Autodesk Fusion 360 part; units mm, degrees
(part 5 of 12)
  line L806 (6.8281, 44.0008) -> (6.6464, 43.7508)
  line L807 (6.8281, 44.3098) -> (6.8281, 44.0008)
  line L808 (6.3475, 43.6553) -> (6.0536, 43.7508)
  line L809 (6.3526, 44.6553) -> (6.6464, 44.5598)
  line L810 (6.3475, 44.6553) -> (6.3526, 44.6553)
  line L811 (6.0536, 44.5598) -> (6.3475, 44.6553)
  line L812 (6.0536, 43.7508) -> (5.8719, 44.0008)
  line L813 (5.8719, 44.3098) -> (6.0536, 44.5598)
  line L814 (6.3475, 41.1153) -> (6.0536, 41.2108)
  line L815 (6.0536, 41.2108) -> (5.8719, 41.4608)
  line L816 (5.8719, 41.4608) -> (5.8719, 41.7698)
  line L817 (5.8719, 41.7698) -> (6.0536, 42.0198)
  line L818 (6.0536, 42.0198) -> (6.3475, 42.1153)
  line L819 (6.3475, 42.1153) -> (6.3526, 42.1153)
  line L820 (6.3526, 42.1153) -> (6.6464, 42.0198)
  line L821 (6.6464, 42.0198) -> (6.8281, 41.7698)
  line L822 (6.8281, 41.7698) -> (6.8281, 41.4608)
  line L823 (6.8281, 41.4608) -> (6.6464, 41.2108)
  line L824 (6.6464, 41.2108) -> (6.3526, 41.1153)
  line L825 (6.3526, 41.1153) -> (6.3475, 41.1153)
  line L826 (5.8719, 39.2298) -> (6.0536, 39.4798)
  line L827 (5.8719, 38.9208) -> (5.8719, 39.2298)
  line L828 (6.3475, 38.5753) -> (6.0536, 38.6708)
  line L829 (6.0536, 39.4798) -> (6.3475, 39.5753)
  line L830 (6.3475, 39.5753) -> (6.3526, 39.5753)
  line L831 (6.3526, 39.5753) -> (6.6464, 39.4798)
  line L832 (6.6464, 39.4798) -> (6.8281, 39.2298)
  line L833 (6.8281, 39.2298) -> (6.8281, 38.9208)
  line L834 (6.8281, 38.9208) -> (6.6464, 38.6708)
  line L835 (6.6464, 38.6708) -> (6.3526, 38.5753)
  line L836 (6.3526, 38.5753) -> (6.3475, 38.5753)
  line L837 (6.0536, 38.6708) -> (5.8719, 38.9208)
  line L838 (23.8336, 39.4798) -> (24.1275, 39.5753)
  line L839 (24.1326, 39.5753) -> (24.4265, 39.4798)
  line L840 (23.8336, 38.6708) -> (23.652, 38.9208)
  line L841 (24.1275, 38.5753) -> (23.8336, 38.6708)
  line L842 (24.4265, 39.4798) -> (24.6081, 39.2298)
  line L843 (24.6081, 39.2298) -> (24.6081, 38.9208)
  line L844 (24.6081, 38.9208) -> (24.4265, 38.6708)
  line L845 (24.4265, 38.6708) -> (24.1326, 38.5753)
  line L846 (24.1326, 38.5753) -> (24.1275, 38.5753)
  line L847 (23.652, 39.2298) -> (23.8336, 39.4798)
  line L848 (24.1275, 39.5753) -> (24.1326, 39.5753)
  line L849 (23.652, 38.9208) -> (23.652, 39.2298)
  line L850 (24.1275, 41.1153) -> (23.8336, 41.2108)
  line L851 (23.8336, 41.2108) -> (23.652, 41.4608)
  line L852 (23.652, 41.4608) -> (23.652, 41.7698)
  line L853 (23.652, 41.7698) -> (23.8336, 42.0198)
  line L854 (23.8336, 42.0198) -> (24.1275, 42.1153)
  line L855 (24.1275, 42.1153) -> (24.1326, 42.1153)
  line L856 (24.1326, 42.1153) -> (24.4265, 42.0198)
  line L857 (24.4265, 42.0198) -> (24.6081, 41.7698)
  line L858 (24.6081, 41.7698) -> (24.6081, 41.4608)
  line L859 (24.6081, 41.4608) -> (24.4265, 41.2108)
  line L860 (24.4265, 41.2108) -> (24.1326, 41.1153)
  line L861 (24.1326, 41.1153) -> (24.1275, 41.1153)
  line L862 (23.652, 43.9292) -> (23.652, 44.2382)
  line L863 (23.652, 44.2382) -> (23.8336, 44.4882)
  line L864 (23.8336, 44.4882) -> (24.1275, 44.5837)
  line L865 (24.1275, 44.5837) -> (24.1326, 44.5837)
  line L866 (24.1326, 44.5837) -> (24.4265, 44.4882)
  line L867 (23.8336, 43.6792) -> (23.652, 43.9292)
  line L868 (24.1275, 43.5837) -> (23.8336, 43.6792)
  line L869 (24.4265, 44.4882) -> (24.6081, 44.2382)
  line L870 (24.6081, 44.2382) -> (24.6081, 43.9292)
  line L871 (24.6081, 43.9292) -> (24.4265, 43.6792)
  line L872 (24.4265, 43.6792) -> (24.1326, 43.5837)
  line L873 (24.1326, 43.5837) -> (24.1275, 43.5837)
  line L874 (24.1275, 46.1953) -> (23.8336, 46.2908)
  line L875 (24.1326, 46.1953) -> (24.1275, 46.1953)
  line L876 (24.4265, 46.2908) -> (24.1326, 46.1953)
  line L877 (24.6081, 46.5408) -> (24.4265, 46.2908)
  line L878 (24.6081, 46.8498) -> (24.6081, 46.5408)
  line L879 (24.4265, 47.0998) -> (24.6081, 46.8498)
  line L880 (24.1326, 47.1953) -> (24.4265, 47.0998)
  line L881 (24.1275, 47.1953) -> (24.1326, 47.1953)
  line L882 (23.8336, 47.0998) -> (24.1275, 47.1953)
  line L883 (23.652, 46.8498) -> (23.8336, 47.0998)
  line L884 (23.652, 46.5408) -> (23.652, 46.8498)
  line L885 (23.8336, 46.2908) -> (23.652, 46.5408)
  line L886 (24.1326, 48.7353) -> (24.1275, 48.7353)
  line L887 (24.1275, 48.7353) -> (23.8336, 48.8308)
  line L888 (23.8336, 48.8308) -> (23.652, 49.0808)
  line L889 (23.652, 49.0808) -> (23.652, 49.3898)
  line L890 (23.652, 49.3898) -> (23.8336, 49.6398)
  line L891 (23.8336, 49.6398) -> (24.1275, 49.7353)
  line L892 (24.1275, 49.7353) -> (24.1326, 49.7353)
  line L893 (24.4265, 49.6398) -> (24.6081, 49.3898)
  line L894 (24.6081, 49.3898) -> (24.6081, 49.0808)
  line L895 (24.6081, 49.0808) -> (24.4265, 48.8308)
  line L896 (24.4265, 48.8308) -> (24.1326, 48.7353)
  line L897 (24.1326, 49.7353) -> (24.4265, 49.6398)
  line L898 (24.1326, 52.2753) -> (24.4265, 52.1798)
  line L899 (24.1275, 51.2753) -> (23.8336, 51.3708)
  line L900 (23.8336, 51.3708) -> (23.652, 51.6208)
  line L901 (23.652, 51.6208) -> (23.652, 51.9298)
  line L902 (23.652, 51.9298) -> (23.8336, 52.1798)
  line L903 (23.8336, 52.1798) -> (24.1275, 52.2753)
  line L904 (24.1275, 52.2753) -> (24.1326, 52.2753)
  line L905 (24.1326, 51.2753) -> (24.1275, 51.2753)
  line L906 (24.4265, 51.3708) -> (24.1326, 51.2753)
  line L907 (24.6081, 51.6208) -> (24.4265, 51.3708)
  line L908 (24.6081, 51.9298) -> (24.6081, 51.6208)
  line L909 (24.4265, 52.1798) -> (24.6081, 51.9298)
  line L910 (24.1326, 53.8153) -> (24.1275, 53.8153)
  line L911 (24.4265, 53.9108) -> (24.1326, 53.8153)
  line L912 (24.6081, 54.1608) -> (24.4265, 53.9108)
  line L913 (24.6081, 54.4698) -> (24.6081, 54.1608)
  line L914 (24.4265, 54.7198) -> (24.6081, 54.4698)
  line L915 (23.652, 54.4698) -> (23.8336, 54.7198)
  line L916 (23.652, 54.1608) -> (23.652, 54.4698)
  line L917 (23.8336, 53.9108) -> (23.652, 54.1608)
  line L918 (24.1275, 53.8153) -> (23.8336, 53.9108)
  line L919 (24.1326, 54.8153) -> (24.4265, 54.7198)
  line L920 (23.8336, 54.7198) -> (24.1275, 54.8153)
  line L921 (24.1275, 54.8153) -> (24.1326, 54.8153)
  line L922 (24.1275, 57.3553) -> (24.1326, 57.3553)
  line L923 (24.1326, 57.3553) -> (24.4265, 57.2598)
  line L924 (23.8336, 57.2598) -> (24.1275, 57.3553)
  line L925 (24.1275, 56.3553) -> (23.8336, 56.4508)
  line L926 (23.8336, 56.4508) -> (23.652, 56.7008)
  line L927 (23.652, 56.7008) -> (23.652, 57.0098)
  line L928 (23.652, 57.0098) -> (23.8336, 57.2598)
  line L929 (24.4265, 57.2598) -> (24.6081, 57.0098)
  line L930 (24.6081, 57.0098) -> (24.6081, 56.7008)
  line L931 (24.6081, 56.7008) -> (24.4265, 56.4508)
  line L932 (24.4265, 56.4508) -> (24.1326, 56.3553)
  line L933 (24.1326, 56.3553) -> (24.1275, 56.3553)
  line L934 (24.1326, 59.8953) -> (24.4265, 59.7998)
  line L935 (23.8336, 58.9908) -> (23.652, 59.2408)
  line L936 (23.652, 59.2408) -> (23.652, 59.5498)
  line L937 (23.652, 59.5498) -> (23.8336, 59.7998)
  line L938 (23.8336, 59.7998) -> (24.1275, 59.8953)
  line L939 (24.1275, 59.8953) -> (24.1326, 59.8953)
  line L940 (24.1275, 58.8953) -> (23.8336, 58.9908)
  line L941 (24.4265, 59.7998) -> (24.6081, 59.5498)
  line L942 (24.6081, 59.5498) -> (24.6081, 59.2408)
  line L943 (24.6081, 59.2408) -> (24.4265, 58.9908)
  line L944 (24.4265, 58.9908) -> (24.1326, 58.8953)
  line L945 (24.1326, 58.8953) -> (24.1275, 58.8953)
  line L946 (24.1275, 61.4353) -> (23.8336, 61.5308)
  line L947 (23.8336, 61.5308) -> (23.652, 61.7808)
  line L948 (23.652, 61.7808) -> (23.652, 62.0898)
  line L949 (23.652, 62.0898) -> (23.8336, 62.3398)
  line L950 (23.8336, 62.3398) -> (24.1275, 62.4353)
  line L951 (24.1275, 62.4353) -> (24.1326, 62.4353)
  line L952 (24.1326, 62.4353) -> (24.4265, 62.3398)
  line L953 (24.4265, 62.3398) -> (24.6081, 62.0898)
  line L954 (24.6081, 62.0898) -> (24.6081, 61.7808)
  line L955 (24.6081, 61.7808) -> (24.4265, 61.5308)
  line L956 (24.4265, 61.5308) -> (24.1326, 61.4353)
  line L957 (24.1326, 61.4353) -> (24.1275, 61.4353)
  line L958 (24.1326, 64.9753) -> (24.4265, 64.8798)
  line L959 (24.1326, 63.9753) -> (24.1275, 63.9753)
  line L960 (24.4265, 64.0708) -> (24.1326, 63.9753)
  line L961 (24.6081, 64.3208) -> (24.4265, 64.0708)
  line L962 (24.6081, 64.6298) -> (24.6081, 64.3208)
  line L963 (24.4265, 64.8798) -> (24.6081, 64.6298)
  line L964 (24.1275, 64.9753) -> (24.1326, 64.9753)
  line L965 (23.8336, 64.8798) -> (24.1275, 64.9753)
  line L966 (23.652, 64.6298) -> (23.8336, 64.8798)
  line L967 (23.652, 64.3208) -> (23.652, 64.6298)
  line L968 (23.8336, 64.0708) -> (23.652, 64.3208)
  line L969 (24.1275, 63.9753) -> (23.8336, 64.0708)
  line L970 (24.1275, 66.5153) -> (23.8336, 66.6108)
  line L971 (23.8336, 66.6108) -> (23.652, 66.8608)
  line L972 (23.652, 66.8608) -> (23.652, 67.1699)
  line L973 (23.652, 67.1699) -> (23.8336, 67.4199)
  line L974 (23.8336, 67.4199) -> (24.1275, 67.5153)
  line L975 (24.1275, 67.5153) -> (24.1326, 67.5153)
  line L976 (24.1326, 67.5153) -> (24.4265, 67.4199)
  line L977 (24.4265, 67.4199) -> (24.6081, 67.1699)
  line L978 (24.6081, 67.1699) -> (24.6081, 66.8608)
  line L979 (24.6081, 66.8608) -> (24.4265, 66.6108)
  line L980 (24.4265, 66.6108) -> (24.1326, 66.5153)
  line L981 (24.1326, 66.5153) -> (24.1275, 66.5153)
  line L982 (23.8336, 69.1508) -> (23.652, 69.4008)
  line L983 (23.652, 69.4008) -> (23.652, 69.7099)
  line L984 (23.652, 69.7099) -> (23.8336, 69.9599)
  line L985 (23.8336, 69.9599) -> (24.1275, 70.0553)
  line L986 (24.1275, 70.0553) -> (24.1326, 70.0553)
  line L987 (24.1326, 69.0553) -> (24.1275, 69.0553)
  line L988 (24.4265, 69.1508) -> (24.1326, 69.0553)
  line L989 (24.6081, 69.4008) -> (24.4265, 69.1508)
  line L990 (24.6081, 69.7099) -> (24.6081, 69.4008)
  line L991 (24.1275, 69.0553) -> (23.8336, 69.1508)
  line L992 (24.4265, 69.9599) -> (24.6081, 69.7099)
  line L993 (24.1326, 70.0553) -> (24.4265, 69.9599)
  line L994 (24.1326, 71.5954) -> (24.1275, 71.5954)
  line L995 (24.4265, 71.6908) -> (24.1326, 71.5954)
  line L996 (24.6081, 71.9408) -> (24.4265, 71.6908)
  line L997 (24.6081, 72.2499) -> (24.6081, 71.9408)
  line L998 (24.4265, 72.4999) -> (24.6081, 72.2499)
  line L999 (24.1326, 72.5954) -> (24.4265, 72.4999)
  line L1000 (24.1275, 72.5954) -> (24.1326, 72.5954)
  line L1001 (23.8336, 72.4999) -> (24.1275, 72.5954)
  line L1002 (23.652, 72.2499) -> (23.8336, 72.4999)
  line L1003 (23.652, 71.9408) -> (23.652, 72.2499)
  line L1004 (23.8336, 71.6908) -> (23.652, 71.9408)
  line L1005 (24.1275, 71.5954) -> (23.8336, 71.6908)
  line L1006 (24.6081, 74.7899) -> (24.6081, 74.4808)
  line L1007 (24.6081, 74.4808) -> (24.4265, 74.2308)
  line L1008 (24.4265, 75.0399) -> (24.6081, 74.7899)
  line L1009 (24.1275, 74.1354) -> (23.8336, 74.2308)
  line L1010 (23.8336, 74.2308) -> (23.652, 74.4808)
  line L1011 (23.652, 74.4808) -> (23.652, 74.7899)
  line L1012 (23.652, 74.7899) -> (23.8336, 75.0399)
  line L1013 (23.8336, 75.0399) -> (24.1275, 75.1354)
  line L1014 (24.1275, 75.1354) -> (24.1326, 75.1354)
  line L1015 (24.1326, 75.1354) -> (24.4265, 75.0399)
  line L1016 (24.4265, 74.2308) -> (24.1326, 74.1354)
  line L1017 (24.1326, 74.1354) -> (24.1275, 74.1354)
  line L1018 (24.1326, 76.6754) -> (24.1275, 76.6754)
  line L1019 (24.1275, 76.6754) -> (23.8336, 76.7709)
  line L1020 (23.8336, 76.7709) -> (23.652, 77.0209)
  line L1021 (23.652, 77.0209) -> (23.652, 77.3299)
  line L1022 (23.652, 77.3299) -> (23.8336, 77.5799)
  line L1023 (23.8336, 77.5799) -> (24.1275, 77.6754)
  line L1024 (24.1275, 77.6754) -> (24.1326, 77.6754)
  line L1025 (24.1326, 77.6754) -> (24.4265, 77.5799)
  line L1026 (24.4265, 77.5799) -> (24.6081, 77.3299)
  line L1027 (24.6081, 77.3299) -> (24.6081, 77.0209)
  line L1028 (24.6081, 77.0209) -> (24.4265, 76.7709)
  line L1029 (24.4265, 76.7709) -> (24.1326, 76.6754)
  line L1030 (24.1326, 79.2154) -> (24.1275, 79.2154)
  line L1031 (24.1275, 79.2154) -> (23.8336, 79.3109)
  line L1032 (23.8336, 79.3109) -> (23.652, 79.5609)
  line L1033 (23.652, 79.5609) -> (23.652, 79.8699)
  line L1034 (23.652, 79.8699) -> (23.8336, 80.1199)
  line L1035 (23.8336, 80.1199) -> (24.1275, 80.2154)
  line L1036 (24.1275, 80.2154) -> (24.1326, 80.2154)
  line L1037 (24.1326, 80.2154) -> (24.4265, 80.1199)
  line L1038 (24.4265, 80.1199) -> (24.6081, 79.8699)
  line L1039 (24.6081, 79.8699) -> (24.6081, 79.5609)
  line L1040 (24.6081, 79.5609) -> (24.4265, 79.3109)
  line L1041 (24.4265, 79.3109) -> (24.1326, 79.2154)
  line L1042 (23.652, 82.1009) -> (23.652, 82.4099)
  line L1043 (24.1275, 81.7554) -> (23.8336, 81.8509)
  line L1044 (23.652, 82.4099) -> (23.8336, 82.6599)
  line L1045 (23.8336, 81.8509) -> (23.652, 82.1009)
  line L1046 (23.8336, 82.6599) -> (24.1275, 82.7554)
  line L1047 (24.1275, 82.7554) -> (24.1326, 82.7554)
  line L1048 (24.1326, 82.7554) -> (24.4265, 82.6599)
  line L1049 (24.4265, 82.6599) -> (24.6081, 82.4099)
  line L1050 (24.6081, 82.4099) -> (24.6081, 82.1009)
  line L1051 (24.6081, 82.1009) -> (24.4265, 81.8509)
  line L1052 (24.4265, 81.8509) -> (24.1326, 81.7554)
  line L1053 (24.1326, 81.7554) -> (24.1275, 81.7554)
  line L1054 (24.1275, 84.2954) -> (23.8336, 84.3909)
  line L1055 (23.8336, 84.3909) -> (23.652, 84.6409)
  line L1056 (23.652, 84.6409) -> (23.652, 84.9499)
  line L1057 (23.652, 84.9499) -> (23.8336, 85.1999)
  line L1058 (23.8336, 85.1999) -> (24.1275, 85.2954)
  line L1059 (24.1275, 85.2954) -> (24.1326, 85.2954)
  line L1060 (24.1326, 85.2954) -> (24.4265, 85.1999)
  line L1061 (24.4265, 85.1999) -> (24.6081, 84.9499)
  line L1062 (24.6081, 84.9499) -> (24.6081, 84.6409)
  line L1063 (24.6081, 84.6409) -> (24.4265, 84.3909)
  line L1064 (24.4265, 84.3909) -> (24.1326, 84.2954)
  line L1065 (24.1326, 84.2954) -> (24.1275, 84.2954)
  line L1066 (24.1326, 87.8354) -> (24.4265, 87.7399)
  line L1067 (24.4265, 87.7399) -> (24.6081, 87.4899)
  line L1068 (24.1275, 86.8354) -> (23.8336, 86.9309)
  line L1069 (23.8336, 86.9309) -> (23.652, 87.1809)
  line L1070 (23.652, 87.1809) -> (23.652, 87.4899)
  line L1071 (23.652, 87.4899) -> (23.8336, 87.7399)
  line L1072 (23.8336, 87.7399) -> (24.1275, 87.8354)
  line L1073 (24.1275, 87.8354) -> (24.1326, 87.8354)
  line L1074 (24.6081, 87.1809) -> (24.4265, 86.9309)
  line L1075 (24.4265, 86.9309) -> (24.1326, 86.8354)
  line L1076 (24.1326, 86.8354) -> (24.1275, 86.8354)
  line L1077 (24.6081, 87.4899) -> (24.6081, 87.1809)
  line L1078 (11.4326, 38.5753) -> (11.4275, 38.5753)
  line L1079 (11.4275, 38.5753) -> (11.1336, 38.6708)
  line L1080 (11.1336, 38.6708) -> (10.952, 38.9208)
  line L1081 (10.952, 38.9208) -> (10.952, 39.2298)
  line L1082 (10.952, 39.2298) -> (11.1336, 39.4798)
  line L1083 (11.1336, 39.4798) -> (11.4275, 39.5753)
  line L1084 (11.4275, 39.5753) -> (11.4326, 39.5753)
  line L1085 (11.4326, 39.5753) -> (11.7265, 39.4798)
  line L1086 (11.7265, 39.4798) -> (11.9081, 39.2298)
  line L1087 (11.9081, 39.2298) -> (11.9081, 38.9208)
  line L1088 (11.9081, 38.9208) -> (11.7265, 38.6708)
  line L1089 (11.7265, 38.6708) -> (11.4326, 38.5753)
  line L1090 (14.2665, 39.4798) -> (14.4481, 39.2298)
  line L1091 (13.9726, 39.5753) -> (14.2665, 39.4798)
  line L1092 (13.9675, 39.5753) -> (13.9726, 39.5753)
  line L1093 (13.6736, 39.4798) -> (13.9675, 39.5753)
  line L1094 (13.492, 39.2298) -> (13.6736, 39.4798)
  line L1095 (13.492, 38.9208) -> (13.492, 39.2298)
  line L1096 (13.6736, 38.6708) -> (13.492, 38.9208)
  line L1097 (13.9675, 38.5753) -> (13.6736, 38.6708)
  line L1098 (14.4481, 39.2298) -> (14.4481, 38.9208)
  line L1099 (14.4481, 38.9208) -> (14.2665, 38.6708)
  line L1100 (14.2665, 38.6708) -> (13.9726, 38.5753)
  line L1101 (13.9726, 38.5753) -> (13.9675, 38.5753)
  line L1102 (16.9881, 39.2298) -> (16.9881, 38.9208)
  line L1103 (16.5075, 38.5753) -> (16.2136, 38.6708)
  line L1104 (16.2136, 38.6708) -> (16.032, 38.9208)
  line L1105 (16.032, 38.9208) -> (16.032, 39.2298)
  line L1106 (16.032, 39.2298) -> (16.2136, 39.4798)
  line L1107 (16.2136, 39.4798) -> (16.5075, 39.5753)
  line L1108 (16.5075, 39.5753) -> (16.5126, 39.5753)
  line L1109 (16.5126, 39.5753) -> (16.8065, 39.4798)
  line L1110 (16.9881, 38.9208) -> (16.8065, 38.6708)
  line L1111 (16.8065, 38.6708) -> (16.5126, 38.5753)
  line L1112 (16.5126, 38.5753) -> (16.5075, 38.5753)
  line L1113 (16.8065, 39.4798) -> (16.9881, 39.2298)
  line L1114 (19.5281, 39.2298) -> (19.5281, 38.9208)
  line L1115 (19.3465, 39.4798) -> (19.5281, 39.2298)
  line L1116 (19.3465, 38.6708) -> (19.0526, 38.5753)
  line L1117 (19.0526, 38.5753) -> (19.0475, 38.5753)
  line L1118 (19.0475, 38.5753) -> (18.7536, 38.6708)
  line L1119 (18.7536, 38.6708) -> (18.572, 38.9208)
  line L1120 (18.572, 38.9208) -> (18.572, 39.2298)
  line L1121 (18.572, 39.2298) -> (18.7536, 39.4798)
  line L1122 (18.7536, 39.4798) -> (19.0475, 39.5753)
  line L1123 (19.0475, 39.5753) -> (19.0526, 39.5753)
  line L1124 (19.0526, 39.5753) -> (19.3465, 39.4798)
  line L1125 (19.5281, 38.9208) -> (19.3465, 38.6708)
  arc A1908 (43.4461, 87.1512) -> (44.9461, 87.1512) centre (44.1961, 87.1512) ccw
  arc A1909 (44.9461, 87.1512) -> (43.4461, 87.1512) centre (44.1961, 87.1512) ccw
  arc A1910 (38.6081, 84.6112) -> (37.084, 84.6112) centre (37.8461, 84.6112) ccw
  arc A1911 (37.084, 84.6112) -> (38.6081, 84.6112) centre (37.8461, 84.6112) ccw
  arc A1912 (74.9461, 87.1512) -> (73.4461, 87.1512) centre (74.1961, 87.1512) ccw
  arc A1913 (73.4461, 87.1512) -> (74.9461, 87.1512) centre (74.1961, 87.1512) ccw
  arc A1914 (67.084, 84.6112) -> (68.6081, 84.6112) centre (67.8461, 84.6112) ccw
  arc A1915 (68.6081, 84.6112) -> (67.084, 84.6112) centre (67.8461, 84.6112) ccw
  arc A1916 (104.9461, 87.1512) -> (103.4461, 87.1512) centre (104.1961, 87.1512) ccw
  arc A1917 (103.4461, 87.1512) -> (104.9461, 87.1512) centre (104.1961, 87.1512) ccw
  arc A1918 (98.6081, 84.6112) -> (97.084, 84.6112) centre (97.8461, 84.6112) ccw
  arc A1919 (97.084, 84.6112) -> (98.6081, 84.6112) centre (97.8461, 84.6112) ccw
  arc A1920 (133.4461, 87.1512) -> (134.9461, 87.1512) centre (134.1961, 87.1512) ccw
  arc A1921 (134.9461, 87.1512) -> (133.4461, 87.1512) centre (134.1961, 87.1512) ccw
  arc A1922 (127.084, 84.6112) -> (128.6081, 84.6112) centre (127.8461, 84.6112) ccw
  arc A1923 (128.6081, 84.6112) -> (127.084, 84.6112) centre (127.8461, 84.6112) ccw
  arc A1924 (163.4461, 87.1512) -> (164.9461, 87.1512) centre (164.1961, 87.1512) ccw
  arc A1925 (164.9461, 87.1512) -> (163.4461, 87.1512) centre (164.1961, 87.1512) ccw
  arc A1926 (157.084, 84.6112) -> (158.6081, 84.6112) centre (157.8461, 84.6112) ccw
  arc A1927 (158.6081, 84.6112) -> (157.084, 84.6112) centre (157.8461, 84.6112) ccw
  arc A1928 (193.4461, 87.1512) -> (194.9461, 87.1512) centre (194.1961, 87.1512) ccw
  arc A1929 (194.9461, 87.1512) -> (193.4461, 87.1512) centre (194.1961, 87.1512) ccw
  arc A1930 (187.084, 84.6112) -> (188.6081, 84.6112) centre (187.8461, 84.6112) ccw
  arc A1931 (188.6081, 84.6112) -> (187.084, 84.6112) centre (187.8461, 84.6112) ccw
  arc A1932 (224.9461, 87.1512) -> (223.4461, 87.1512) centre (224.1961, 87.1512) ccw
  arc A1933 (223.4461, 87.1512) -> (224.9461, 87.1512) centre (224.1961, 87.1512) ccw
  arc A1934 (217.084, 84.6112) -> (218.6081, 84.6112) centre (217.8461, 84.6112) ccw
  arc A1935 (218.6081, 84.6112) -> (217.084, 84.6112) centre (217.8461, 84.6112) ccw
  arc A1936 (43.4461, 57.1512) -> (44.9461, 57.1512) centre (44.1961, 57.1512) ccw
  arc A1937 (44.9461, 57.1512) -> (43.4461, 57.1512) centre (44.1961, 57.1512) ccw
  arc A1938 (37.084, 54.6112) -> (38.6081, 54.6112) centre (37.8461, 54.6112) ccw
  arc A1939 (38.6081, 54.6112) -> (37.084, 54.6112) centre (37.8461, 54.6112) ccw
  arc A1940 (73.4461, 57.1512) -> (74.9461, 57.1512) centre (74.1961, 57.1512) ccw
  arc A1941 (74.9461, 57.1512) -> (73.4461, 57.1512) centre (74.1961, 57.1512) ccw
  arc A1942 (67.084, 54.6112) -> (68.6081, 54.6112) centre (67.8461, 54.6112) ccw
  arc A1943 (68.6081, 54.6112) -> (67.084, 54.6112) centre (67.8461, 54.6112) ccw
  arc A1944 (103.4461, 57.1512) -> (104.9461, 57.1512) centre (104.1961, 57.1512) ccw
  arc A1945 (104.9461, 57.1512) -> (103.4461, 57.1512) centre (104.1961, 57.1512) ccw
  arc A1946 (97.084, 54.6112) -> (98.6081, 54.6112) centre (97.8461, 54.6112) ccw
  arc A1947 (98.6081, 54.6112) -> (97.084, 54.6112) centre (97.8461, 54.6112) ccw
  arc A1948 (134.9461, 57.1512) -> (133.4461, 57.1512) centre (134.1961, 57.1512) ccw
  arc A1949 (133.4461, 57.1512) -> (134.9461, 57.1512) centre (134.1961, 57.1512) ccw
  arc A1950 (127.084, 54.6112) -> (128.6081, 54.6112) centre (127.8461, 54.6112) ccw
  arc A1951 (128.6081, 54.6112) -> (127.084, 54.6112) centre (127.8461, 54.6112) ccw
  arc A1952 (163.4461, 57.1512) -> (164.9461, 57.1512) centre (164.1961, 57.1512) ccw
  arc A1953 (164.9461, 57.1512) -> (163.4461, 57.1512) centre (164.1961, 57.1512) ccw
  arc A1954 (157.084, 54.6112) -> (158.6081, 54.6112) centre (157.8461, 54.6112) ccw
  arc A1955 (158.6081, 54.6112) -> (157.084, 54.6112) centre (157.8461, 54.6112) ccw
  arc A1956 (193.4461, 57.1512) -> (194.9461, 57.1512) centre (194.1961, 57.1512) ccw
  arc A1957 (194.9461, 57.1512) -> (193.4461, 57.1512) centre (194.1961, 57.1512) ccw
  arc A1958 (187.084, 54.6112) -> (188.6081, 54.6112) centre (187.8461, 54.6112) ccw
  arc A1959 (188.6081, 54.6112) -> (187.084, 54.6112) centre (187.8461, 54.6112) ccw
  arc A1960 (223.4461, 57.1512) -> (224.9461, 57.1512) centre (224.1961, 57.1512) ccw
  arc A1961 (224.9461, 57.1512) -> (223.4461, 57.1512) centre (224.1961, 57.1512) ccw
  arc A1962 (218.6081, 54.6112) -> (217.084, 54.6112) centre (217.8461, 54.6112) ccw
  arc A1963 (217.084, 54.6112) -> (218.6081, 54.6112) centre (217.8461, 54.6112) ccw
  arc A1964 (44.9461, 27.1512) -> (43.4461, 27.1512) centre (44.1961, 27.1512) ccw
  arc A1965 (43.4461, 27.1512) -> (44.9461, 27.1512) centre (44.1961, 27.1512) ccw
  arc A1966 (38.6081, 24.6112) -> (37.084, 24.6112) centre (37.8461, 24.6112) ccw
  arc A1967 (37.084, 24.6112) -> (38.6081, 24.6112) centre (37.8461, 24.6112) ccw
  arc A1968 (81.0294, 27.2071) -> (79.5294, 27.2071) centre (80.2794, 27.2071) ccw
  arc A1969 (79.5294, 27.2071) -> (81.0294, 27.2071) centre (80.2794, 27.2071) ccw
  arc A1970 (73.1674, 24.6671) -> (74.6914, 24.6671) centre (73.9294, 24.6671) ccw
  arc A1971 (74.6914, 24.6671) -> (73.1674, 24.6671) centre (73.9294, 24.6671) ccw
  arc A1972 (109.5294, 27.2071) -> (111.0294, 27.2071) centre (110.2794, 27.2071) ccw
  arc A1973 (111.0294, 27.2071) -> (109.5294, 27.2071) centre (110.2794, 27.2071) ccw
  arc A1974 (103.1674, 24.6671) -> (104.6914, 24.6671) centre (103.9294, 24.6671) ccw
  arc A1975 (104.6914, 24.6671) -> (103.1674, 24.6671) centre (103.9294, 24.6671) ccw
  arc A1976 (139.5294, 27.2071) -> (141.0294, 27.2071) centre (140.2794, 27.2071) ccw
  arc A1977 (141.0294, 27.2071) -> (139.5294, 27.2071) centre (140.2794, 27.2071) ccw
  arc A1978 (133.1674, 24.6671) -> (134.6914, 24.6671) centre (133.9294, 24.6671) ccw
  arc A1979 (134.6914, 24.6671) -> (133.1674, 24.6671) centre (133.9294, 24.6671) ccw
  arc A1980 (169.5294, 27.2071) -> (171.0294, 27.2071) centre (170.2794, 27.2071) ccw
  arc A1981 (171.0294, 27.2071) -> (169.5294, 27.2071) centre (170.2794, 27.2071) ccw
  arc A1982 (163.1674, 24.6671) -> (164.6914, 24.6671) centre (163.9294, 24.6671) ccw
  arc A1983 (164.6914, 24.6671) -> (163.1674, 24.6671) centre (163.9294, 24.6671) ccw
  arc A1984 (199.5294, 27.2071) -> (201.0294, 27.2071) centre (200.2794, 27.2071) ccw
  arc A1985 (201.0294, 27.2071) -> (199.5294, 27.2071) centre (200.2794, 27.2071) ccw
  arc A1986 (193.1674, 24.6671) -> (194.6914, 24.6671) centre (193.9294, 24.6671) ccw
  arc A1987 (194.6914, 24.6671) -> (193.1674, 24.6671) centre (193.9294, 24.6671) ccw
  arc A1988 (119.7492, -60.2389) -> (118.2492, -60.2389) centre (118.9992, -60.2389) ccw
  arc A1989 (118.2492, -60.2389) -> (119.7492, -60.2389) centre (118.9992, -60.2389) ccw
  arc A1990 (111.8872, -62.7789) -> (113.4112, -62.7789) centre (112.6492, -62.7789) ccw
  arc A1991 (113.4112, -62.7789) -> (111.8872, -62.7789) centre (112.6492, -62.7789) ccw
  arc A1992 (44.9461, -2.8488) -> (43.4461, -2.8488) centre (44.1961, -2.8488) ccw
  arc A1993 (43.4461, -2.8488) -> (44.9461, -2.8488) centre (44.1961, -2.8488) ccw
  arc A1994 (38.6081, -5.3888) -> (37.084, -5.3888) centre (37.8461, -5.3888) ccw
  arc A1995 (37.084, -5.3888) -> (38.6081, -5.3888) centre (37.8461, -5.3888) ccw
  arc A1996 (91.9514, -2.8919) -> (90.4514, -2.8919) centre (91.2014, -2.8919) ccw
  arc A1997 (90.4514, -2.8919) -> (91.9514, -2.8919) centre (91.2014, -2.8919) ccw
  arc A1998 (85.6134, -5.432) -> (84.0894, -5.432) centre (84.8514, -5.432) ccw
  arc A1999 (84.0894, -5.432) -> (85.6134, -5.432) centre (84.8514, -5.432) ccw
  arc A2000 (120.4514, -2.8919) -> (121.9514, -2.8919) centre (121.2014, -2.8919) ccw
  arc A2001 (121.9514, -2.8919) -> (120.4514, -2.8919) centre (121.2014, -2.8919) ccw
  arc A2002 (114.0894, -5.432) -> (115.6134, -5.432) centre (114.8514, -5.432) ccw
  arc A2003 (115.6134, -5.432) -> (114.0894, -5.432) centre (114.8514, -5.432) ccw
  arc A2004 (150.4514, -2.8919) -> (151.9514, -2.8919) centre (151.2014, -2.8919) ccw
  arc A2005 (151.9514, -2.8919) -> (150.4514, -2.8919) centre (151.2014, -2.8919) ccw
  arc A2006 (144.0894, -5.432) -> (145.6134, -5.432) centre (144.8514, -5.432) ccw
  arc A2007 (145.6134, -5.432) -> (144.0894, -5.432) centre (144.8514, -5.432) ccw
  arc A2008 (180.4514, -2.8919) -> (181.9514, -2.8919) centre (181.2014, -2.8919) ccw
  arc A2009 (181.9514, -2.8919) -> (180.4514, -2.8919) centre (181.2014, -2.8919) ccw
  arc A2010 (174.0894, -5.432) -> (175.6134, -5.432) centre (174.8514, -5.432) ccw
  arc A2011 (175.6134, -5.432) -> (174.0894, -5.432) centre (174.8514, -5.432) ccw
  arc A2012 (210.4514, -2.8919) -> (211.9514, -2.8919) centre (211.2014, -2.8919) ccw
  arc A2013 (211.9514, -2.8919) -> (210.4514, -2.8919) centre (211.2014, -2.8919) ccw
  arc A2014 (204.0894, -5.432) -> (205.6134, -5.432) centre (204.8514, -5.432) ccw
  arc A2015 (205.6134, -5.432) -> (204.0894, -5.432) centre (204.8514, -5.432) ccw
  arc A2016 (162.3183, -60.2389) -> (163.8183, -60.2389) centre (163.0683, -60.2389) ccw
  arc A2017 (163.8183, -60.2389) -> (162.3183, -60.2389) centre (163.0683, -60.2389) ccw
  arc A2018 (155.9563, -62.7789) -> (157.4803, -62.7789) centre (156.7183, -62.7789) ccw
  arc A2019 (157.4803, -62.7789) -> (155.9563, -62.7789) centre (156.7183, -62.7789) ccw
  arc A2020 (44.9461, -32.8488) -> (43.4461, -32.8488) centre (44.1961, -32.8488) ccw
  arc A2021 (43.4461, -32.8488) -> (44.9461, -32.8488) centre (44.1961, -32.8488) ccw
  arc A2022 (37.084, -35.3888) -> (38.6081, -35.3888) centre (37.8461, -35.3888) ccw
  arc A2023 (38.6081, -35.3888) -> (37.084, -35.3888) centre (37.8461, -35.3888) ccw
  arc A2024 (99.9764, -32.864) -> (101.4764, -32.864) centre (100.7264, -32.864) ccw
  arc A2025 (101.4764, -32.864) -> (99.9764, -32.864) centre (100.7264, -32.864) ccw
  arc A2026 (93.6144, -35.404) -> (95.1384, -35.404) centre (94.3764, -35.404) ccw
  arc A2027 (95.1384, -35.404) -> (93.6144, -35.404) centre (94.3764, -35.404) ccw
  arc A2028 (18.981, -44.6179) -> (19.8811, -44.6179) centre (19.431, -44.6179) ccw
  arc A2029 (19.8811, -44.6179) -> (18.981, -44.6179) centre (19.431, -44.6179) ccw
  arc A2030 (18.981, -42.0779) -> (19.8811, -42.0779) centre (19.431, -42.0779) ccw
  arc A2031 (19.8811, -42.0779) -> (18.981, -42.0779) centre (19.431, -42.0779) ccw
  arc A2032 (18.981, -39.5379) -> (19.8811, -39.5379) centre (19.431, -39.5379) ccw
  arc A2033 (19.8811, -39.5379) -> (18.981, -39.5379) centre (19.431, -39.5379) ccw
  arc A2034 (18.981, -36.9979) -> (19.8811, -36.9979) centre (19.431, -36.9979) ccw
  arc A2035 (19.8811, -36.9979) -> (18.981, -36.9979) centre (19.431, -36.9979) ccw
  arc A2036 (18.981, -34.4579) -> (19.8811, -34.4579) centre (19.431, -34.4579) ccw
  arc A2037 (19.8811, -34.4579) -> (18.981, -34.4579) centre (19.431, -34.4579) ccw
  arc A2038 (18.981, -31.9179) -> (19.8811, -31.9179) centre (19.431, -31.9179) ccw
  arc A2039 (19.8811, -31.9179) -> (18.981, -31.9179) centre (19.431, -31.9179) ccw
  arc A2040 (18.981, -29.3779) -> (19.8811, -29.3779) centre (19.431, -29.3779) ccw
  arc A2041 (19.8811, -29.3779) -> (18.981, -29.3779) centre (19.431, -29.3779) ccw
  arc A2042 (18.981, -26.8378) -> (19.8811, -26.8378) centre (19.431, -26.8378) ccw
  arc A2043 (19.8811, -26.8378) -> (18.981, -26.8378) centre (19.431, -26.8378) ccw
  arc A2044 (18.981, -24.2978) -> (19.8811, -24.2978) centre (19.431, -24.2978) ccw
  arc A2045 (19.8811, -24.2978) -> (18.981, -24.2978) centre (19.431, -24.2978) ccw
  arc A2046 (18.981, -21.7578) -> (19.8811, -21.7578) centre (19.431, -21.7578) ccw
  arc A2047 (19.8811, -21.7578) -> (18.981, -21.7578) centre (19.431, -21.7578) ccw
  arc A2048 (18.981, -19.2178) -> (19.8811, -19.2178) centre (19.431, -19.2178) ccw
  arc A2049 (19.8811, -19.2178) -> (18.981, -19.2178) centre (19.431, -19.2178) ccw
  arc A2050 (19.8811, -16.6778) -> (18.981, -16.6778) centre (19.431, -16.6778) ccw
  arc A2051 (18.981, -16.6778) -> (19.8811, -16.6778) centre (19.431, -16.6778) ccw
  arc A2052 (19.8811, -14.1378) -> (18.981, -14.1378) centre (19.431, -14.1378) ccw
  arc A2053 (18.981, -14.1378) -> (19.8811, -14.1378) centre (19.431, -14.1378) ccw
  arc A2054 (19.8811, -11.5978) -> (18.981, -11.5978) centre (19.431, -11.5978) ccw
  arc A2055 (18.981, -11.5978) -> (19.8811, -11.5978) centre (19.431, -11.5978) ccw
  arc A2056 (11.361, -44.6179) -> (12.261, -44.6179) centre (11.811, -44.6179) ccw
  arc A2057 (12.261, -44.6179) -> (11.361, -44.6179) centre (11.811, -44.6179) ccw
  arc A2058 (11.361, -42.0779) -> (12.261, -42.0779) centre (11.811, -42.0779) ccw
  arc A2059 (12.261, -42.0779) -> (11.361, -42.0779) centre (11.811, -42.0779) ccw
  arc A2060 (11.361, -39.5379) -> (12.261, -39.5379) centre (11.811, -39.5379) ccw
  arc A2061 (12.261, -39.5379) -> (11.361, -39.5379) centre (11.811, -39.5379) ccw
  arc A2062 (11.361, -36.9979) -> (12.261, -36.9979) centre (11.811, -36.9979) ccw
  arc A2063 (12.261, -36.9979) -> (11.361, -36.9979) centre (11.811, -36.9979) ccw
  arc A2064 (11.361, -34.4579) -> (12.261, -34.4579) centre (11.811, -34.4579) ccw
  arc A2065 (12.261, -34.4579) -> (11.361, -34.4579) centre (11.811, -34.4579) ccw
  arc A2066 (11.361, -31.9179) -> (12.261, -31.9179) centre (11.811, -31.9179) ccw
  arc A2067 (12.261, -31.9179) -> (11.361, -31.9179) centre (11.811, -31.9179) ccw
  arc A2068 (11.361, -29.3779) -> (12.261, -29.3779) centre (11.811, -29.3779) ccw
  arc A2069 (12.261, -29.3779) -> (11.361, -29.3779) centre (11.811, -29.3779) ccw
  arc A2070 (12.261, -26.8378) -> (11.361, -26.8378) centre (11.811, -26.8378) ccw
  arc A2071 (11.361, -26.8378) -> (12.261, -26.8378) centre (11.811, -26.8378) ccw
  arc A2072 (11.361, -24.2978) -> (12.261, -24.2978) centre (11.811, -24.2978) ccw
  arc A2073 (12.261, -24.2978) -> (11.361, -24.2978) centre (11.811, -24.2978) ccw
  arc A2074 (11.361, -21.7578) -> (12.261, -21.7578) centre (11.811, -21.7578) ccw
  arc A2075 (12.261, -21.7578) -> (11.361, -21.7578) centre (11.811, -21.7578) ccw
  arc A2076 (11.361, -19.2178) -> (12.261, -19.2178) centre (11.811, -19.2178) ccw
  arc A2077 (12.261, -19.2178) -> (11.361, -19.2178) centre (11.811, -19.2178) ccw
  arc A2078 (11.361, -16.6778) -> (12.261, -16.6778) centre (11.811, -16.6778) ccw
  arc A2079 (12.261, -16.6778) -> (11.361, -16.6778) centre (11.811, -16.6778) ccw
  arc A2080 (11.361, -14.1378) -> (12.261, -14.1378) centre (11.811, -14.1378) ccw
  arc A2081 (12.261, -14.1378) -> (11.361, -14.1378) centre (11.811, -14.1378) ccw
  arc A2082 (11.361, -11.5978) -> (12.261, -11.5978) centre (11.811, -11.5978) ccw
  arc A2083 (12.261, -11.5978) -> (11.361, -11.5978) centre (11.811, -11.5978) ccw
  arc A2084 (217.7364, 4.7852) -> (218.6364, 4.7852) centre (218.1864, 4.7852) ccw
  arc A2085 (218.6364, 4.7852) -> (217.7364, 4.7852) centre (218.1864, 4.7852) ccw
  arc A2086 (217.7364, 7.3252) -> (218.6364, 7.3252) centre (218.1864, 7.3252) ccw
  arc A2087 (218.6364, 7.3252) -> (217.7364, 7.3252) centre (218.1864, 7.3252) ccw
  arc A2088 (217.7364, 9.8652) -> (218.6364, 9.8652) centre (218.1864, 9.8652) ccw
  arc A2089 (218.6364, 9.8652) -> (217.7364, 9.8652) centre (218.1864, 9.8652) ccw
  arc A2090 (218.6364, 12.4052) -> (217.7364, 12.4052) centre (218.1864, 12.4052) ccw
  arc A2091 (217.7364, 12.4052) -> (218.6364, 12.4052) centre (218.1864, 12.4052) ccw
  arc A2092 (217.7364, 14.9452) -> (218.6364, 14.9452) centre (218.1864, 14.9452) ccw
  arc A2093 (218.6364, 14.9452) -> (217.7364, 14.9452) centre (218.1864, 14.9452) ccw
  arc A2094 (217.7364, 17.4852) -> (218.6364, 17.4852) centre (218.1864, 17.4852) ccw
  arc A2095 (218.6364, 17.4852) -> (217.7364, 17.4852) centre (218.1864, 17.4852) ccw
  arc A2096 (217.7364, 20.0252) -> (218.6364, 20.0252) centre (218.1864, 20.0252) ccw
  arc A2097 (218.6364, 20.0252) -> (217.7364, 20.0252) centre (218.1864, 20.0252) ccw
  arc A2098 (217.7364, 22.5653) -> (218.6364, 22.5653) centre (218.1864, 22.5653) ccw
  arc A2099 (218.6364, 22.5653) -> (217.7364, 22.5653) centre (218.1864, 22.5653) ccw
  arc A2100 (217.7364, 25.1053) -> (218.6364, 25.1053) centre (218.1864, 25.1053) ccw
  arc A2101 (218.6364, 25.1053) -> (217.7364, 25.1053) centre (218.1864, 25.1053) ccw
  arc A2102 (217.7364, 27.6453) -> (218.6364, 27.6453) centre (218.1864, 27.6453) ccw
  arc A2103 (218.6364, 27.6453) -> (217.7364, 27.6453) centre (218.1864, 27.6453) ccw
  arc A2104 (218.6364, 30.1853) -> (217.7364, 30.1853) centre (218.1864, 30.1853) ccw
  arc A2105 (217.7364, 30.1853) -> (218.6364, 30.1853) centre (218.1864, 30.1853) ccw
  arc A2106 (217.7364, 32.7253) -> (218.6364, 32.7253) centre (218.1864, 32.7253) ccw
  arc A2107 (218.6364, 32.7253) -> (217.7364, 32.7253) centre (218.1864, 32.7253) ccw
  arc A2108 (217.7364, 35.2653) -> (218.6364, 35.2653) centre (218.1864, 35.2653) ccw
  arc A2109 (218.6364, 35.2653) -> (217.7364, 35.2653) centre (218.1864, 35.2653) ccw
  arc A2110 (217.7364, 37.8053) -> (218.6364, 37.8053) centre (218.1864, 37.8053) ccw
  arc A2111 (218.6364, 37.8053) -> (217.7364, 37.8053) centre (218.1864, 37.8053) ccw
  arc A2112 (210.1164, 4.7852) -> (211.0164, 4.7852) centre (210.5664, 4.7852) ccw
  arc A2113 (211.0164, 4.7852) -> (210.1164, 4.7852) centre (210.5664, 4.7852) ccw
  arc A2114 (210.1164, 7.3252) -> (211.0164, 7.3252) centre (210.5664, 7.3252) ccw
  arc A2115 (211.0164, 7.3252) -> (210.1164, 7.3252) centre (210.5664, 7.3252) ccw
  arc A2116 (210.1164, 9.8652) -> (211.0164, 9.8652) centre (210.5664, 9.8652) ccw
  arc A2117 (211.0164, 9.8652) -> (210.1164, 9.8652) centre (210.5664, 9.8652) ccw
  arc A2118 (210.1164, 12.4052) -> (211.0164, 12.4052) centre (210.5664, 12.4052) ccw
  arc A2119 (211.0164, 12.4052) -> (210.1164, 12.4052) centre (210.5664, 12.4052) ccw
  arc A2120 (211.0164, 14.9452) -> (210.1164, 14.9452) centre (210.5664, 14.9452) ccw
  arc A2121 (210.1164, 14.9452) -> (211.0164, 14.9452) centre (210.5664, 14.9452) ccw
  arc A2122 (210.1164, 17.4852) -> (211.0164, 17.4852) centre (210.5664, 17.4852) ccw
  arc A2123 (211.0164, 17.4852) -> (210.1164, 17.4852) centre (210.5664, 17.4852) ccw
  arc A2124 (210.1164, 20.0252) -> (211.0164, 20.0252) centre (210.5664, 20.0252) ccw
  arc A2125 (211.0164, 20.0252) -> (210.1164, 20.0252) centre (210.5664, 20.0252) ccw
  arc A2126 (210.1164, 22.5653) -> (211.0164, 22.5653) centre (210.5664, 22.5653) ccw
  arc A2127 (211.0164, 22.5653) -> (210.1164, 22.5653) centre (210.5664, 22.5653) ccw
  arc A2128 (210.1164, 25.1053) -> (211.0164, 25.1053) centre (210.5664, 25.1053) ccw
  arc A2129 (211.0164, 25.1053) -> (210.1164, 25.1053) centre (210.5664, 25.1053) ccw
  arc A2130 (210.1164, 27.6453) -> (211.0164, 27.6453) centre (210.5664, 27.6453) ccw
  arc A2131 (211.0164, 27.6453) -> (210.1164, 27.6453) centre (210.5664, 27.6453) ccw
  arc A2132 (210.1164, 30.1853) -> (211.0164, 30.1853) centre (210.5664, 30.1853) ccw
  arc A2133 (211.0164, 30.1853) -> (210.1164, 30.1853) centre (210.5664, 30.1853) ccw
  arc A2134 (211.0164, 32.7253) -> (210.1164, 32.7253) centre (210.5664, 32.7253) ccw
  arc A2135 (210.1164, 32.7253) -> (211.0164, 32.7253) centre (210.5664, 32.7253) ccw
  arc A2136 (210.1164, 35.2653) -> (211.0164, 35.2653) centre (210.5664, 35.2653) ccw
  arc A2137 (211.0164, 35.2653) -> (210.1164, 35.2653) centre (210.5664, 35.2653) ccw
  arc A2138 (210.1164, 37.8053) -> (211.0164, 37.8053) centre (210.5664, 37.8053) ccw
  arc A2139 (211.0164, 37.8053) -> (210.1164, 37.8053) centre (210.5664, 37.8053) ccw
  arc A2140 (129.9764, -32.864) -> (131.4764, -32.864) centre (130.7264, -32.864) ccw
  arc A2141 (131.4764, -32.864) -> (129.9764, -32.864) centre (130.7264, -32.864) ccw
  arc A2142 (123.6144, -35.404) -> (125.1384, -35.404) centre (124.3764, -35.404) ccw
  arc A2143 (125.1384, -35.404) -> (123.6144, -35.404) centre (124.3764, -35.404) ccw
  arc A2144 (159.9764, -32.864) -> (161.4764, -32.864) centre (160.7264, -32.864) ccw
  arc A2145 (161.4764, -32.864) -> (159.9764, -32.864) centre (160.7264, -32.864) ccw
  arc A2146 (153.6144, -35.404) -> (155.1384, -35.404) centre (154.3764, -35.404) ccw
  arc A2147 (155.1384, -35.404) -> (153.6144, -35.404) centre (154.3764, -35.404) ccw
  arc A2148 (189.9764, -32.864) -> (191.4764, -32.864) centre (190.7264, -32.864) ccw
  arc A2149 (191.4764, -32.864) -> (189.9764, -32.864) centre (190.7264, -32.864) ccw
  arc A2150 (185.1384, -35.404) -> (183.6144, -35.404) centre (184.3764, -35.404) ccw
  arc A2151 (183.6144, -35.404) -> (185.1384, -35.404) centre (184.3764, -35.404) ccw
  arc A2152 (221.4764, -32.864) -> (219.9764, -32.864) centre (220.7264, -32.864) ccw
  arc A2153 (219.9764, -32.864) -> (221.4764, -32.864) centre (220.7264, -32.864) ccw
  arc A2154 (215.1384, -35.404) -> (213.6144, -35.404) centre (214.3764, -35.404) ccw
  arc A2155 (213.6144, -35.404) -> (215.1384, -35.404) centre (214.3764, -35.404) ccw
  arc A2156 (208.2684, -60.2389) -> (206.7684, -60.2389) centre (207.5184, -60.2389) ccw
  arc A2157 (206.7684, -60.2389) -> (208.2684, -60.2389) centre (207.5184, -60.2389) ccw
  arc A2158 (200.4064, -62.7789) -> (201.9304, -62.7789) centre (201.1684, -62.7789) ccw
  arc A2159 (201.9304, -62.7789) -> (200.4064, -62.7789) centre (201.1684, -62.7789) ccw
  arc A2160 (43.4461, -60.2389) -> (44.9461, -60.2389) centre (44.1961, -60.2389) ccw
  arc A2161 (44.9461, -60.2389) -> (43.4461, -60.2389) centre (44.1961, -60.2389) ccw
  arc A2162 (37.084, -62.7789) -> (38.6081, -62.7789) centre (37.8461, -62.7789) ccw
  arc A2163 (38.6081, -62.7789) -> (37.084, -62.7789) centre (37.8461, -62.7789) ccw
  arc A2164 (77.6091, -60.2389) -> (79.1091, -60.2389) centre (78.3591, -60.2389) ccw
  arc A2165 (79.1091, -60.2389) -> (77.6091, -60.2389) centre (78.3591, -60.2389) ccw
  arc A2166 (71.2471, -62.7789) -> (72.7711, -62.7789) centre (72.0091, -62.7789) ccw
  arc A2167 (72.7711, -62.7789) -> (71.2471, -62.7789) centre (72.0091, -62.7789) ccw
  arc A2168 (16.822, -2.3268) -> (17.722, -2.3268) centre (17.272, -2.3268) ccw
  arc A2169 (17.722, -2.3268) -> (16.822, -2.3268) centre (17.272, -2.3268) ccw
  arc A2170 (16.822, 0.2132) -> (17.722, 0.2132) centre (17.272, 0.2132) ccw
  arc A2171 (17.722, 0.2132) -> (16.822, 0.2132) centre (17.272, 0.2132) ccw
  arc A2172 (16.822, 2.7532) -> (17.722, 2.7532) centre (17.272, 2.7532) ccw
  arc A2173 (17.722, 2.7532) -> (16.822, 2.7532) centre (17.272, 2.7532) ccw
  arc A2174 (16.822, 5.2932) -> (17.722, 5.2932) centre (17.272, 5.2932) ccw
  arc A2175 (17.722, 5.2932) -> (16.822, 5.2932) centre (17.272, 5.2932) ccw
  arc A2176 (16.822, 7.8332) -> (17.722, 7.8332) centre (17.272, 7.8332) ccw
  arc A2177 (17.722, 7.8332) -> (16.822, 7.8332) centre (17.272, 7.8332) ccw
  arc A2178 (16.822, 10.3732) -> (17.722, 10.3732) centre (17.272, 10.3732) ccw
  arc A2179 (17.722, 10.3732) -> (16.822, 10.3732) centre (17.272, 10.3732) ccw
  arc A2180 (16.822, 12.9132) -> (17.722, 12.9132) centre (17.272, 12.9132) ccw
  arc A2181 (17.722, 12.9132) -> (16.822, 12.9132) centre (17.272, 12.9132) ccw
  arc A2182 (16.822, 15.4532) -> (17.722, 15.4532) centre (17.272, 15.4532) ccw
  arc A2183 (17.722, 15.4532) -> (16.822, 15.4532) centre (17.272, 15.4532) ccw
  arc A2184 (17.722, 17.9932) -> (16.822, 17.9932) centre (17.272, 17.9932) ccw
  arc A2185 (16.822, 17.9932) -> (17.722, 17.9932) centre (17.272, 17.9932) ccw
  arc A2186 (16.822, 20.5332) -> (17.722, 20.5332) centre (17.272, 20.5332) ccw
  arc A2187 (17.722, 20.5332) -> (16.822, 20.5332) centre (17.272, 20.5332) ccw
  arc A2188 (16.822, 23.0733) -> (17.722, 23.0733) centre (17.272, 23.0733) ccw
  arc A2189 (17.722, 23.0733) -> (16.822, 23.0733) centre (17.272, 23.0733) ccw
  arc A2190 (16.822, 25.6133) -> (17.722, 25.6133) centre (17.272, 25.6133) ccw
  arc A2191 (17.722, 25.6133) -> (16.822, 25.6133) centre (17.272, 25.6133) ccw
  arc A2192 (16.822, 28.1533) -> (17.722, 28.1533) centre (17.272, 28.1533) ccw
  arc A2193 (17.722, 28.1533) -> (16.822, 28.1533) centre (17.272, 28.1533) ccw
  arc A2194 (16.822, 30.6933) -> (17.722, 30.6933) centre (17.272, 30.6933) ccw
  arc A2195 (17.722, 30.6933) -> (16.822, 30.6933) centre (17.272, 30.6933) ccw
  arc A2196 (10.102, -2.3268) -> (9.202, -2.3268) centre (9.652, -2.3268) ccw
  arc A2197 (9.202, -2.3268) -> (10.102, -2.3268) centre (9.652, -2.3268) ccw
  arc A2198 (9.202, 0.2132) -> (10.102, 0.2132) centre (9.652, 0.2132) ccw
  arc A2199 (10.102, 0.2132) -> (9.202, 0.2132) centre (9.652, 0.2132) ccw
  arc A2200 (9.202, 2.7532) -> (10.102, 2.7532) centre (9.652, 2.7532) ccw
  arc A2201 (10.102, 2.7532) -> (9.202, 2.7532) centre (9.652, 2.7532) ccw
  arc A2202 (9.202, 5.2932) -> (10.102, 5.2932) centre (9.652, 5.2932) ccw
  arc A2203 (10.102, 5.2932) -> (9.202, 5.2932) centre (9.652, 5.2932) ccw
  arc A2204 (9.202, 7.8332) -> (10.102, 7.8332) centre (9.652, 7.8332) ccw
  arc A2205 (10.102, 7.8332) -> (9.202, 7.8332) centre (9.652, 7.8332) ccw
  arc A2206 (9.202, 10.3732) -> (10.102, 10.3732) centre (9.652, 10.3732) ccw
  arc A2207 (10.102, 10.3732) -> (9.202, 10.3732) centre (9.652, 10.3732) ccw
  arc A2208 (9.202, 12.9132) -> (10.102, 12.9132) centre (9.652, 12.9132) ccw
  arc A2209 (10.102, 12.9132) -> (9.202, 12.9132) centre (9.652, 12.9132) ccw
  arc A2210 (9.202, 15.4532) -> (10.102, 15.4532) centre (9.652, 15.4532) ccw
  arc A2211 (10.102, 15.4532) -> (9.202, 15.4532) centre (9.652, 15.4532) ccw
  arc A2212 (10.102, 17.9932) -> (9.202, 17.9932) centre (9.652, 17.9932) ccw
  arc A2213 (9.202, 17.9932) -> (10.102, 17.9932) centre (9.652, 17.9932) ccw
  arc A2214 (9.202, 20.5332) -> (10.102, 20.5332) centre (9.652, 20.5332) ccw
  arc A2215 (10.102, 20.5332) -> (9.202, 20.5332) centre (9.652, 20.5332) ccw
  arc A2216 (9.202, 23.0733) -> (10.102, 23.0733) centre (9.652, 23.0733) ccw
  arc A2217 (10.102, 23.0733) -> (9.202, 23.0733) centre (9.652, 23.0733) ccw
  arc A2218 (9.202, 25.6133) -> (10.102, 25.6133) centre (9.652, 25.6133) ccw
  arc A2219 (10.102, 25.6133) -> (9.202, 25.6133) centre (9.652, 25.6133) ccw
  arc A2220 (10.102, 28.1533) -> (9.202, 28.1533) centre (9.652, 28.1533) ccw
  arc A2221 (9.202, 28.1533) -> (10.102, 28.1533) centre (9.652, 28.1533) ccw
  arc A2222 (9.202, 30.6933) -> (10.102, 30.6933) centre (9.652, 30.6933) ccw
  arc A2223 (10.102, 30.6933) -> (9.202, 30.6933) centre (9.652, 30.6933) ccw
  line L1126 (209.4522, 77.9041) -> (209.2272, 77.7406)
  line L1127 (209.5381, 78.1686) -> (209.4522, 77.9041)
  line L1128 (208.9491, 77.7406) -> (208.724, 77.9041)
  line L1129 (208.724, 77.9041) -> (208.6381, 78.1686)
  line L1130 (208.6381, 78.1686) -> (208.6381, 79.0686)
  line L1131 (208.6381, 79.0686) -> (208.724, 79.3331)
  line L1132 (208.724, 79.3331) -> (208.9491, 79.4965)
  line L1133 (208.9491, 79.4965) -> (209.2272, 79.4965)
  line L1134 (209.2272, 79.4965) -> (209.4522, 79.3331)
  line L1135 (209.4522, 79.3331) -> (209.5381, 79.0686)
  line L1136 (209.5381, 79.0686) -> (209.5381, 78.1686)
  line L1137 (209.2272, 77.7406) -> (208.9491, 77.7406)
  line L1138 (205.1288, 78.0689) -> (205.1288, 77.1688)
  line L1139 (205.1288, 77.1688) -> (205.0429, 76.9042)
  line L1140 (205.0429, 76.9042) -> (204.8179, 76.7408)
  line L1141 (204.8179, 76.7408) -> (204.5397, 76.7408)
  line L1142 (204.5397, 76.7408) -> (204.3147, 76.9042)
  line L1143 (204.3147, 76.9042) -> (204.2288, 77.1688)
  line L1144 (204.2288, 77.1688) -> (204.2288, 78.0689)
  line L1145 (204.2288, 78.0689) -> (204.3147, 78.3334)
  line L1146 (204.3147, 78.3334) -> (204.5397, 78.4969)
  line L1147 (204.5397, 78.4969) -> (204.8179, 78.4969)
  line L1148 (204.8179, 78.4969) -> (205.0429, 78.3334)
  line L1149 (205.0429, 78.3334) -> (205.1288, 78.0689)
  line L1150 (209.5381, 83.0686) -> (209.5381, 82.1686)
  line L1151 (209.5381, 82.1686) -> (209.4522, 81.9041)
  line L1152 (209.4522, 81.9041) -> (209.2272, 81.7406)
  line L1153 (209.2272, 81.7406) -> (208.9491, 81.7406)
  line L1154 (208.9491, 81.7406) -> (208.724, 81.9041)
  line L1155 (208.724, 81.9041) -> (208.6381, 82.1686)
  line L1156 (208.6381, 82.1686) -> (208.6381, 83.0686)
  line L1157 (208.6381, 83.0686) -> (208.724, 83.3331)
  line L1158 (208.724, 83.3331) -> (208.9491, 83.4965)
  line L1159 (208.9491, 83.4965) -> (209.2272, 83.4965)
  line L1160 (209.2272, 83.4965) -> (209.4522, 83.3331)
  line L1161 (209.4522, 83.3331) -> (209.5381, 83.0686)
  line L1162 (209.5383, 85.5076) -> (209.4523, 85.2431)
  line L1163 (209.5383, 86.4078) -> (209.5383, 85.5076)
  line L1164 (209.4523, 85.2431) -> (209.2273, 85.0796)
  line L1165 (209.2273, 85.0796) -> (208.9492, 85.0796)
  line L1166 (208.9492, 85.0796) -> (208.7242, 85.2431)
  line L1167 (208.7242, 85.2431) -> (208.6382, 85.5076)
  line L1168 (208.6382, 85.5076) -> (208.6382, 86.4078)
  line L1169 (208.6382, 86.4078) -> (208.7242, 86.6723)
  line L1170 (208.7242, 86.6723) -> (208.9492, 86.8358)
  line L1171 (208.9492, 86.8358) -> (209.2273, 86.8358)
  line L1172 (209.2273, 86.8358) -> (209.4523, 86.6723)
  line L1173 (209.4523, 86.6723) -> (209.5383, 86.4078)
  arc A2224 (15.9168, -58.0817) -> (16.2218, -58.0817) centre (16.0693, -58.0817) ccw
  arc A2225 (16.2218, -58.0817) -> (15.9168, -58.0817) centre (16.0693, -58.0817) ccw
  arc A2226 (9.3745, -32.9778) -> (9.0695, -32.9778) centre (9.222, -32.9778) ccw
  arc A2227 (9.0695, -32.9778) -> (9.3745, -32.9778) centre (9.222, -32.9778) ccw
  arc A2228 (212.0695, 39.9996) -> (212.3745, 39.9996) centre (212.222, 39.9996) ccw
  arc A2229 (212.3745, 39.9996) -> (212.0695, 39.9996) centre (212.222, 39.9996) ccw
  arc A2230 (38.6468, -70.5666) -> (38.9518, -70.5666) centre (38.7993, -70.5666) ccw
  arc A2231 (38.9518, -70.5666) -> (38.6468, -70.5666) centre (38.7993, -70.5666) ccw
  arc A2232 (79.7202, -71.3265) -> (80.0252, -71.3265) centre (79.8727, -71.3265) ccw
  arc A2233 (80.0252, -71.3265) -> (79.7202, -71.3265) centre (79.8727, -71.3265) ccw
  arc A2234 (73.4688, -54.9445) -> (73.7738, -54.9445) centre (73.6213, -54.9445) ccw
  arc A2235 (73.7738, -54.9445) -> (73.4688, -54.9445) centre (73.6213, -54.9445) ccw
  arc A2236 (198.6057, -67.6341) -> (198.9107, -67.6341) centre (198.7582, -67.6341) ccw
  arc A2237 (198.9107, -67.6341) -> (198.6057, -67.6341) centre (198.7582, -67.6341) ccw
  arc A2238 (46.8373, -67.6341) -> (47.1423, -67.6341) centre (46.9898, -67.6341) ccw
  arc A2239 (47.1423, -67.6341) -> (46.8373, -67.6341) centre (46.9898, -67.6341) ccw
  arc A2240 (216.6481, 25.5439) -> (216.9531, 25.5439) centre (216.8006, 25.5439) ccw
  arc A2241 (216.9531, 25.5439) -> (216.6481, 25.5439) centre (216.8006, 25.5439) ccw
  arc A2242 (40.6049, -31.2036) -> (40.9099, -31.2036) centre (40.7574, -31.2036) ccw
  arc A2243 (40.9099, -31.2036) -> (40.6049, -31.2036) centre (40.7574, -31.2036) ccw
  arc A2244 (18.5219, 22.7108) -> (18.8269, 22.7108) centre (18.6744, 22.7108) ccw
  arc A2245 (18.8269, 22.7108) -> (18.5219, 22.7108) centre (18.6744, 22.7108) ccw
  arc A2246 (155.417, -41.9994) -> (155.722, -41.9994) centre (155.5695, -41.9994) ccw
  arc A2247 (155.722, -41.9994) -> (155.417, -41.9994) centre (155.5695, -41.9994) ccw
  arc A2248 (189.99, -40.1378) -> (190.295, -40.1378) centre (190.1425, -40.1378) ccw
  arc A2249 (190.295, -40.1378) -> (189.99, -40.1378) centre (190.1425, -40.1378) ccw
  arc A2250 (125.3771, -43.2072) -> (125.6821, -43.2072) centre (125.5296, -43.2072) ccw
  arc A2251 (125.6821, -43.2072) -> (125.3771, -43.2072) centre (125.5296, -43.2072) ccw
  arc A2252 (155.6268, -39.6346) -> (155.9318, -39.6346) centre (155.7793, -39.6346) ccw
  arc A2253 (155.9318, -39.6346) -> (155.6268, -39.6346) centre (155.7793, -39.6346) ccw
  arc A2254 (182.549, -14.2681) -> (182.8541, -14.2681) centre (182.7015, -14.2681) ccw
  arc A2255 (182.8541, -14.2681) -> (182.549, -14.2681) centre (182.7015, -14.2681) ccw
  arc A2256 (131.7619, -30.2935) -> (132.0669, -30.2935) centre (131.9144, -30.2935) ccw
  arc A2257 (132.0669, -30.2935) -> (131.7619, -30.2935) centre (131.9144, -30.2935) ccw
  arc A2258 (16.4297, -59.686) -> (16.7347, -59.686) centre (16.5822, -59.686) ccw
  arc A2259 (16.7347, -59.686) -> (16.4297, -59.686) centre (16.5822, -59.686) ccw
  arc A2260 (214.5813, 38.2495) -> (214.8863, 38.2495) centre (214.7338, 38.2495) ccw
  arc A2261 (214.8863, 38.2495) -> (214.5813, 38.2495) centre (214.7338, 38.2495) ccw
  arc A2262 (15.7809, -1.528) -> (15.4759, -1.528) centre (15.6284, -1.528) ccw
  arc A2263 (15.4759, -1.528) -> (15.7809, -1.528) centre (15.6284, -1.528) ccw
  arc A2264 (133.8078, 19.914) -> (133.5028, 19.914) centre (133.6553, 19.914) ccw
  arc A2265 (133.5028, 19.914) -> (133.8078, 19.914) centre (133.6553, 19.914) ccw
  arc A2266 (38.4563, -41.9862) -> (38.7613, -41.9862) centre (38.6088, -41.9862) ccw
  arc A2267 (38.7613, -41.9862) -> (38.4563, -41.9862) centre (38.6088, -41.9862) ccw
  arc A2268 (96.0604, -39.4411) -> (96.3654, -39.4411) centre (96.2129, -39.4411) ccw